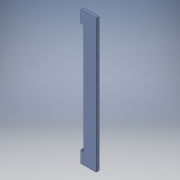
# Autodesk Inventor part: EBF_001.1-side-plate_cup-holder
Saved by Autodesk Inventor 2019 (Build 230136000, 136)
## iProperties
Created: 2019-02-28
Part Number: EBF_001.1-side-plate_cup-holder
Material: Generic
Document SubType Name: Modeling
Designer: Rene
Density: 1 g/cm^3
Appearance: Rubber - Blue
Author: Rene
Autodesk Inventor part; units mm, degrees
ref_plane "YZ Plane" through (0, 0, 0) normal (1, 0, 0) x (0, 1, 0)
ref_plane "XZ Plane" through (0, 0, 0) normal (0, 1, 0) x (-1, 0, 0)
ref_plane "XY Plane" through (0, 0, 0) normal (0, 0, 1) x (1, 0, 0)
sketch "Sketch1" plane through (0, 0, 0) normal (0, 0, 1) x (1, 0, 0)
  line L0 (-10, -110) -> (10, -110)
  line L1 (10, -110) -> (10, 110)
  line L2 (10, 110) -> (-10, 110)
  line L3 (-10, 110) -> (-10, -110)
  point P0 (0, 0)
  dimension "width" = 20
  dimension "d1" = 10
  dimension "d2" = 220
  dimension "d3" = 110
  constraints: 8 end point, 2 parallel, 1 horizontal, 1 perpendicular
  measures "width" distance of L0.start L0.end
  measures "d1" horizontal distance of point (0, 0) L0.start
  measures "d2" distance of L2.end L0.start
  measures "d3" vertical distance of point (0, 0) L0.start
extrude "Extrusion1" add sketch "Sketch1" along normal blind 5
sketch "Sketch4" plane through (-10, -110, 0) normal (-1, 0, 0) x (0, 0, 1)
  line L0 (5, 0) -> (5, 220) projected
  line L1 (0, 0) -> (5, 0)
  line L2 (5, 0) -> (5, 19.8)
  line L3 (5, 19.8) -> (0, 19.8)
  line L4 (0, 19.8) -> (0, 0)
  point P0 (0, 110)
  dimension "d29" = 19.8
  constraints: 8 end point, 2 parallel, 1 horizontal, 1 perpendicular, 1 point on line
  measures "d29" distance between parallel lines of L1 L3
extrude "Extrusion4" add sketch "Sketch4" along normal blind 5
mirror "Mirror1" about plane through (0, 0, 0) normal (0, 1, 0) of "Extrusion4"
equation "\"d1\" = 0.5 * width"
equation "\"d3\" = 0.5 * d2"
body "Solid1"
